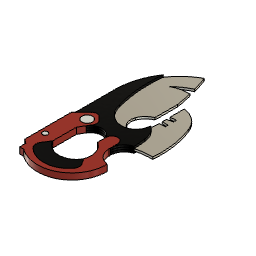
ジェーン_武器_mk1 v1 (Autodesk Fusion 360 design; units mm, degrees)
Autodesk Fusion 360 part; units mm, degrees
sketch "スケッチ1" plane through (0, 0, 0) normal (0, 0, 1) x (1, 0, 0)
  line L0 (0, 0) -> (0, 155) construction
  line L1 (0, 15) -> (0, 60)
  line L2 (0, 60) -> (9.8995, 69.8995)
  line L3 (15, 27) -> (15, 50)
  line L4 (15, 50) -> (21, 60)
  line L5 (17, 70) -> (21, 66)
  arc A0 (17, 70) -> (9.8995, 69.8995) centre (13.4986, 66.4986) ccw
  arc A1 (21, 60) -> (21, 66) centre (16, 63) ccw
  circle A2 centre (13.4285, 62.0062) radius 5
  arc A3 (15, 27) -> (45, 27) centre (30, 34.9444) ccw
  arc A4 (10.3023, 19.7727) -> (11, 12) centre (16.8203, 16.4401) ccw
  line L6 (15, 27) -> (10.3023, 19.7727)
  arc A5 (11, 12) -> (48.5115, 14.8863) centre (28.5562, 29.033) ccw
  arc A6 (48.5115, 14.8863) -> (48.5115, 21.726) centre (43.1372, 18.3062) ccw
  arc A7 (48.5115, 21.726) -> (45, 27) centre (-80.5305, -60.3874) ccw
  arc A8 (45, 27) -> (44.5546, 40.2891) centre (27.5338, 33.0666) ccw
  arc A9 (44.5546, 40.2891) -> (37.9047, 47.4813) centre (30.2489, 33.7325) ccw
  line L7 (37.9047, 47.4813) -> (37.9047, 56)
  arc A10 (37.9047, 56) -> (18.6, 56) centre (28.2523, 50.2086) ccw
  arc A11 (49, 56) -> (37.9047, 56) centre (43.4523, 56) ccw
  line L8 (49, 56) -> (49, 47.4813)
  arc A12 (49, 47.4813) -> (61, 34) centre (62.5728, 47.4813) ccw
  arc A13 (8, 6) -> (61, 34) centre (27.5906, 33.0786) ccw
  line L9 (8, 6) -> (4, 6)
  line L10 (4, 6) -> (4, 12)
  line L11 (4, 12) -> (0, 15)
  line L12 (2, 62) -> (2, 100)
  arc A14 (13.1919, 136.048) -> (2, 100) centre (65.6493, 100) ccw
  arc A15 (13.1919, 136.048) -> (17, 90) centre (130.1571, 122.5393) ccw
  arc A16 (17, 90) -> (30, 74) centre (38.9146, 94.5244) ccw
  arc A17 (30, 74) -> (41, 74) centre (35.5, 91.1601) ccw
  arc A18 (41, 74) -> (48.1072, 80.4137) centre (35.5062, 87.2324) ccw
  arc A19 (48.1072, 80.4137) -> (49.865, 87.2324) centre (35.2739, 87.3581) ccw
  arc A20 (58.1149, 73.1401) -> (49.865, 87.2324) centre (38.7249, 71.2499) ccw
  arc A21 (59, 62) -> (58.1149, 73.1401) centre (-252.7239, 42.8372) ccw
  arc A22 (59, 62) -> (49, 49) centre (62.45, 49) ccw
  arc A23 (34, 155) -> (13.1919, 136.048) centre (64.7476, 100.3422) ccw
  arc A24 (38.4403, 141.1292) -> (34, 155) centre (-87.582, 108.4337) ccw
  arc A25 (38.4403, 141.1292) -> (24.2063, 131.3639) centre (61.4881, 92.2782) ccw
  arc A26 (40, 135) -> (24.2063, 131.3639) centre (40.4754, 96.8171) ccw
  arc A27 (43, 120) -> (40, 135) centre (-170.2438, 85.1512) ccw
  line L13 (43, 120) -> (43, 98.083)
  arc A28 (43, 98.083) -> (33.5663, 88.4851) centre (49.1342, 82.6187) ccw
  arc A29 (33.5663, 88.4851) -> (35.5, 77.8074) centre (43.8523, 84.8339) ccw
  arc A30 (35.5, 77.8074) -> (43.478, 75.3274) centre (41.4552, 82.8926) ccw
  line L14 (49.865, 87.2324) -> (49.9322, 95.031)
  line L15 (49.9322, 95.031) -> (55.5377, 95.7143)
  line L16 (55.5377, 95.7143) -> (55.5589, 98.1814)
  line L17 (55.5589, 98.1814) -> (49.9322, 98.2299)
  line L18 (49.9322, 98.2299) -> (49.9647, 102.0012)
  line L19 (49.9647, 102.0012) -> (55.5698, 103.5114)
  line L20 (55.5698, 103.5114) -> (55.5932, 106.229)
  line L21 (55.5932, 106.229) -> (49.9484, 105.6745)
  line L22 (49.9484, 105.6745) -> (49.9484, 119.5817)
  arc A31 (69, 105) -> (49.9484, 119.5817) centre (47.2483, 96.3173) ccw
  arc A32 (75, 64) -> (69, 105) centre (-13.8176, 71.9413) ccw
  arc A33 (75, 64) -> (59, 62) centre (74.3596, 4.1233) ccw
  circle A34 centre (4.9497, 29.8728) radius 2.5
  dimension "d5" = 155
  dimension "d6" = 45
  dimension "d7" = 15
  dimension "d8" = 135
  dimension "d9" = 14
  dimension "d10" = 10
  dimension "d11" = 5
  constraint coincident L0.start origin
  constraint vertical L0
  constraint coincident L0 L1.start
  constraint coincident L0 L1.end
  constraint parallel L0 L3
  constraint tangent L5 A0
  constraint tangent L4 A1
  constraint tangent A6 A7
  constraint tangent A3 A9
  constraint vertical L7
  constraint tangent L4 A10
  constraint coincident L4 A10.end
  constraint tangent L7 A11
  constraint tangent A11 L8
  constraint parallel L0 L8
  constraint equal L7 L8
  constraint tangent L8 A12
  constraint tangent A11 A13
  constraint perpendicular L1 L9
  constraint perpendicular L9 L10
  constraint coincident L2 L12.start
  constraint parallel L10 L12
  constraint tangent L12 A14
  constraint tangent A15 A17
  constraint tangent A16 A18
  constraint tangent A18 A19
  constraint tangent A20 A21
  constraint tangent L8 A22
  constraint coincident L8 A22.end
  constraint tangent A23 A25
  constraint tangent A23 A26
  constraint tangent A24 A27
  constraint vertical L13
  constraint tangent A17 A30
  constraint coincident A18 A30.end
  constraint tangent A19 L14
  constraint parallel L14 L16
  constraint perpendicular L14 L17
  constraint perpendicular L17 L18
  constraint parallel L18 L20
  constraint tangent A31 A32
  constraint tangent A22 A33
  measures "d5" distance of L0.start L0.end
  measures "d6" distance of L1.start L1.end
  measures "d7" distance of L0.start L1.start
  measures "d8" angle of L1 L2
  measures "d9" distance of L1.end L2.end
  measures "d10" diameter of A2
  measures "d11" diameter of A34
extrude "押し出し1" add sketch "スケッチ1" along normal blind 2 contours L2 L4 L5 A0 A1 A10 A11 L8 L12 A14 A15 A16 A17 A18 A19 A20 A21 A22 makes body 1
extrude "押し出し2" add sketch "スケッチ1" along normal blind 6 separate body contours A3 A4 L6 A5 A6 A7 makes body 2
extrude "押し出し3" add sketch "スケッチ1" along normal blind 6 separate body contours L1 L2 L3 L4 L5 A0 A1 A4 L6 A5 A6 A7 A8 A9 L7 A11 L8 A12 A13 L9 L10 L11 makes body 3
extrude "押し出し4" add sketch "スケッチ1" along normal blind 6 separate body contours A2 | A34 makes body 4 at (18.4223, 61.757, 4) makes body 5 at (7.4466, 29.7482, 4)
extrude "押し出し5" add sketch "スケッチ1" along normal blind 2 separate body contours L2 L4 L5 A0 A1 A10 A11 L8 L12 A14 A15 A16 A17 A18 A19 A20 A21 A22 | A15 A16 A17 A18 A23 A24 A25 A26 A27 L13 A28 A29 A30 | A20 A21 L14 L15 L16 L17 L18 L19 L20 L21 L22 A31 A32 A33 makes body 6
move_body "移動1" bodies 6 to x (1, 0, 0) y (0, 1, 0) z (0, 0, 1) at (0, 0, 2)
extrude "押し出し6" add sketch "スケッチ1" along normal blind 2 separate body contours L2 L4 L5 A0 A1 A10 A11 L8 L12 A14 A15 A16 A17 A18 A19 A20 A21 A22 makes body 7
move_body "移動2" bodies 7 to x (1, 0, 0) y (0, 1, 0) z (0, 0, 1) at (0, 0, 4)
